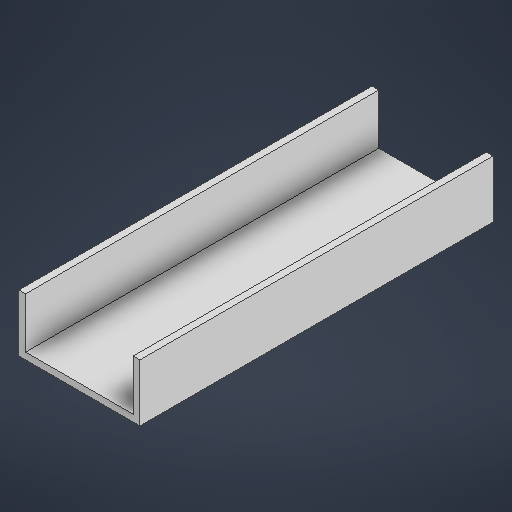
# Autodesk Inventor part: inslide
Saved by Autodesk Inventor 2026.2 (Build 302298000, 298)
## iProperties
Created: 2026-02-23
Part Number: inslide
Material: Generic
Document SubType Name: Sheet Metal
Designer: danda
Density: 1 g/cm^3
Sheet Metal Rule: Default_mm
Appearance: Default
Author: danda
Autodesk Inventor part; units mm, degrees
ref_plane "YZ Plane" through (0, 0, 0) normal (1, 0, 0) x (0, 1, 0)
ref_plane "XZ Plane" through (0, 0, 0) normal (0, 1, 0) x (-1, 0, 0)
ref_plane "XY Plane" through (0, 0, 0) normal (0, 0, 1) x (1, 0, 0)
sketch "Sketch1" plane through (0, 0, 0) normal (0, 0, 1) x (1, 0, 0)
  line L0 (10.7104, 9.7791) -> (42.7104, 9.7791)
  line L1 (42.7104, 9.7791) -> (42.7104, 24.7791)
  line L2 (10.7104, 9.7791) -> (10.7104, 24.7791)
  line L3 (8.7104, 24.7791) -> (8.7104, 7.7791)
  line L4 (8.7104, 7.7791) -> (44.7104, 7.7791)
  line L5 (44.7104, 7.7791) -> (44.7104, 24.7791)
  line L6 (8.7104, 24.7791) -> (10.7104, 24.7791)
  line L7 (42.7104, 24.7791) -> (44.7104, 24.7791)
  point P0 (0, 0)
  dimension "d0" = 32
  dimension "d1" = 15
  dimension "d2" = 15
  dimension "d3" = 2
  constraints: 16 end point, 3 horizontal, 2 perpendicular, 1 vertical, 2 other
  measures "d0" distance of L0.start L0.end
  measures "d1" distance of L0.end L1.end
  measures "d2" distance of L0.start L2.end
  measures "d3" distance between parallel lines of L2 L3
extrude "Extrusion1" add sketch "Sketch1" along normal blind 100 and the other way blind 5
sketch "Sketch2" plane through (8.7104, 7.7791, -5) normal (0, -1, 0) x (1, 0, 0)
  circle A0 centre (30.17, 93.8) radius 2.5
  line L0 (36, 0) -> (36, 105) projected
  line L1 (0, 105) -> (36, 105) projected
  point P0 (-8.7104, 5)
  dimension "d6" = 5
  dimension "d7" = 5.83
  dimension "d8" = 11.2
  constraints: 1 centre point
  measures "d6" diameter of A0
  measures "d7" distance from line of L0 A0.centre
  measures "d8" distance from line of L1 A0.centre
extrude "Extrusion2" cut sketch "Sketch2" against normal blind 2
equation "\"BendRadius\" = Thickness"
equation "\"BendReliefWidth\" = Thickness"
equation "\"BendReliefDepth\" = 0.5 * Thickness"
equation "\"CornerReliefSize\" = 4 * Thickness"
equation "\"MinimumRemnant\" = 2 * Thickness"
equation "\"TransitionRadius\" = BendRadius"
equation "\"JacobiRadiusSize\" = BendRadius"
equation "\"GapSize\" = Thickness"
equation "\"Thickness\" = 0.5"
body "Solid1"
